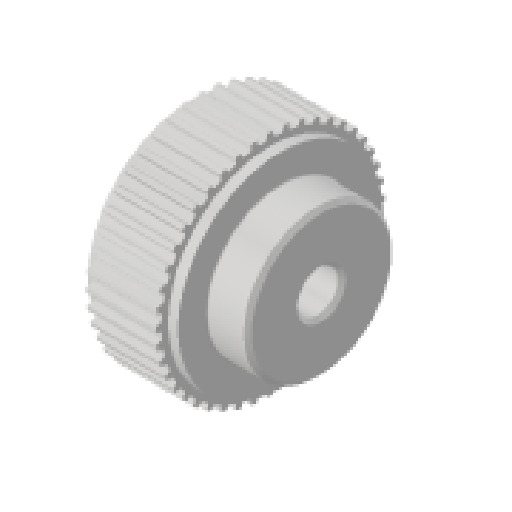
# Autodesk Inventor part: 4202514444
Saved by Autodesk Inventor 2025.1 (Build 291241000, 241)
## iProperties
Category: PARTsolutions
Company: CHIARAVALLI
Created: 2025-04-22
Part Number: 4202514444
Material: Generic
Catalog Web Link: www.cadenas.de
Description: MXL 025 BODY-Timing pulleys with pilot bore
Vendor: CHIARAVALLI
Document SubType Name: Modeling
Designer: psAdmin
Manufacturer: CHIARAVALLI
Mass: 7.09327 g
Surface Area: 28.8164 cm^2
Volume: 7.09327 cm^3
Density: 1 g/cm^3
Appearance: PSOLRGB-175-175-175
PSOL_IDENT_0: {$CADENAS_DATA/23d-libs/chiaravalli/open_transmission/toothed_pulleys/timing_pulleys_with_pilot_bore
PSOL_IDENT_1: /mxl/mxl_025_aluminium.prj},167 {VTYP=3D},{NB=4202514444},{LINA=4202514444},{NN=MXL 025 BODY},{DATE=
PSOL_IDENT_2: 05.08.2024 16:01:07},{GEOMDATE=30.04.2024 10:20:00},{VERSION=},{LINEID=120},{WBVAR=},{WBNUMERIC=}  {
PSOL_IDENT_3: NB=4202514444},{LINA=4202514444},{KT=DUMMY},{CODE=42025144},{TYPE=44 MXL 025},{T=44},{EXEC=1F},{DP=2
PSOL_IDENT_4: 8.46},{DE=27.95},{DF=36},{DM=18},{DM1=-},{F=11.0},{L=16},{D=5},{NF=510},{WEIGHT=0.03},{MAT=Aluminium
PSOL_IDENT_5: 6082-T6},{DX=5},{NFX=510},{DM1X=0.0},{L1=25.0}
NB: 4202514444
NN: MXL 025 BODY
NT: Timing pulleys with pilot bore
NBSYN: $CODE.$T.
LINA: 4202514444
CATALOG: Chiaravalli
CODE: 42025144
T: 44
EXEC: 1F
DP: 28.46
DE: 27.95
DF: 36
DM: 18
DM1: -
F: 11
L: 16
D: 5
NF: 510
WEIGHT: 0.03
MAT: Aluminium 6082-T6
DX: 5
NFX: 510
DM1X: 0
L1: 25
SUPPLIER: CHIARAVALLI
ARTICLENO: 4202514444
BOMINFO: 4202514444
CREATOR: CADENAS GmbH
Title: 4202514444
Author: Cadenas PARTsolutions
Comments: Timing pulleys with pilot bore
Autodesk Inventor part; units mm, degrees
sketch "Sketch_5" plane through (0, 0, 0) normal (0, 0, 1) x (1, 0, 0)
  line L0 (16, 0) -> (0, 0)
  line L1 (0, 3) -> (0.5, 2.5)
  line L2 (0.5, 2.5) -> (15.5, 2.5)
  line L3 (15.5, 2.5) -> (16, 3)
  line L4 (16, 3) -> (16, 8.5)
  line L5 (16, 8.5) -> (15.5, 9)
  line L6 (15.5, 9) -> (11.2, 9)
  arc A0 (11, 9.2) -> (11.2, 9) centre (11.2, 9.2) ccw
  line L7 (11, 9.2) -> (11, 12.5)
  line L8 (11, 12.5) -> (9.75, 12.5)
  line L9 (9.75, 12.5) -> (9.75, 16.77)
  line L10 (9.75, 16.77) -> (1.25, 16.77)
  line L11 (1.25, 16.77) -> (1.25, 12.5)
  line L12 (1.25, 12.5) -> (0, 12.5)
  line L13 (0, 12.5) -> (0, 3)
  constraints: 28 end point, 2 point on circle, 1 centre point
revolve "Revolution1" add sketch "Sketch_5" angle 360 about axis through (16, 0, 0) along (1, 0, 0)
sketch "Sketch_3" plane through (1.25, 0, 0) normal (1, 0, 0) x (0, 0, -1)
  line L0 (-27.95, 27.95) -> (-27.95, -27.95)
  line L1 (-27.95, -27.95) -> (27.95, -27.95)
  line L2 (27.95, -27.95) -> (27.95, 27.95)
  line L3 (27.95, 27.95) -> (-27.95, 27.95)
  arc A0 (-13.973, 0.2355) -> (-13.973, -0.2355) centre (0, 0) ccw
  arc A1 (-13.973, -0.2355) -> (-13.8923, -0.3319) centre (-13.873, -0.2338) ccw
  line L4 (-13.8923, -0.3319) -> (-13.509, -0.4073)
  arc A2 (-13.2673, -0.6862) -> (-13.509, -0.4073) centre (-13.5669, -0.7016) ccw
  arc A3 (-13.2673, -0.6862) -> (-13.2299, -1.209) centre (0, 0) ccw
  arc A4 (-13.4295, -1.5194) -> (-13.2299, -1.209) centre (-13.5286, -1.2363) ccw
  line L5 (-13.4295, -1.5194) -> (-13.7982, -1.6485)
  arc A5 (-13.7982, -1.6485) -> (-13.8643, -1.7555) centre (-13.7651, -1.7429) ccw
  arc A6 (-13.8643, -1.7555) -> (-13.7973, -2.2217) centre (0, 0) ccw
  arc A7 (-13.7973, -2.2217) -> (-13.7037, -2.3056) centre (-13.6985, -2.2058) ccw
  line L6 (-13.7037, -2.3056) -> (-13.3135, -2.3257)
  arc A8 (-13.0346, -2.5673) -> (-13.3135, -2.3257) centre (-13.3289, -2.6253) ccw
  arc A9 (-13.0346, -2.5673) -> (-12.9232, -3.0795) centre (0, 0) ccw
  arc A10 (-13.0765, -3.4151) -> (-12.9232, -3.0795) centre (-13.215, -3.149) ccw
  line L7 (-13.0765, -3.4151) -> (-13.4231, -3.5954)
  arc A11 (-13.4231, -3.5954) -> (-13.4734, -3.7107) centre (-13.3769, -3.6841) ccw
  arc A12 (-13.4734, -3.7107) -> (-13.3407, -4.1626) centre (0, 0) ccw
  arc A13 (-13.3407, -4.1626) -> (-13.2361, -4.2324) centre (-13.2452, -4.1328) ccw
  line L8 (-13.2361, -4.2324) -> (-12.847, -4.1967)
  arc A14 (-12.5365, -4.3962) -> (-12.847, -4.1967) centre (-12.8196, -4.4955) ccw
  arc A15 (-12.5365, -4.3962) -> (-12.3534, -4.8873) centre (0, 0) ccw
  arc A16 (-12.4574, -5.2414) -> (-12.3534, -4.8873) centre (-12.6323, -4.9976) ccw
  line L9 (-12.4574, -5.2414) -> (-12.7748, -5.4691)
  arc A17 (-12.7748, -5.4691) -> (-12.8081, -5.5904) centre (-12.7165, -5.5504) ccw
  arc A18 (-12.8081, -5.5904) -> (-12.6125, -6.0188) centre (0, 0) ccw
  arc A19 (-12.6125, -6.0188) -> (-12.499, -6.073) centre (-12.5222, -5.9757) ccw
  line L10 (-12.499, -6.073) -> (-12.119, -5.9823)
  arc A20 (-11.7833, -6.1356) -> (-12.119, -5.9823) centre (-12.0494, -6.2741) ccw
  arc A21 (-11.7833, -6.1356) -> (-11.5321, -6.5956) centre (0, 0) ccw
  arc A22 (-11.5847, -6.9609) -> (-11.5321, -6.5956) centre (-11.7925, -6.7445) ccw
  line L11 (-11.5847, -6.9609) -> (-11.8664, -7.2315)
  arc A23 (-11.8664, -7.2315) -> (-11.8822, -7.3563) centre (-11.7971, -7.3036) ccw
  arc A24 (-11.8822, -7.3563) -> (-11.6275, -7.7525) centre (0, 0) ccw
  arc A25 (-11.6275, -7.7525) -> (-11.5075, -7.79) centre (-11.5443, -7.697) ccw
  line L12 (-11.5075, -7.79) -> (-11.1443, -7.6461)
  arc A26 (-10.7902, -7.7501) -> (-11.1443, -7.6461) centre (-11.0338, -7.9251) ccw
  arc A27 (-10.7902, -7.7501) -> (-10.4761, -8.1697) centre (0, 0) ccw
  arc A28 (-10.4761, -8.5387) -> (-10.4761, -8.1697) centre (-10.7126, -8.3541) ccw
  line L13 (-10.4761, -8.5387) -> (-10.7165, -8.8467)
  arc A29 (-10.7165, -8.8467) -> (-10.7143, -8.9724) centre (-10.6376, -8.9082) ccw
  arc A30 (-10.7143, -8.9724) -> (-10.4059, -9.3284) centre (0, 0) ccw
  arc A31 (-10.4059, -9.3284) -> (-10.2817, -9.3484) centre (-10.3314, -9.2616) ccw
  line L14 (-10.2817, -9.3484) -> (-9.9427, -9.1543)
  arc A32 (-9.5774, -9.2068) -> (-9.9427, -9.1543) centre (-9.7937, -9.4147) ccw
  arc A33 (-9.5774, -9.2068) -> (-9.2068, -9.5774) centre (0, 0) ccw
  arc A34 (-9.1543, -9.9427) -> (-9.2068, -9.5774) centre (-9.4147, -9.7937) ccw
  line L15 (-9.1543, -9.9427) -> (-9.3484, -10.2817)
  arc A35 (-9.3484, -10.2817) -> (-9.3284, -10.4059) centre (-9.2616, -10.3314) ccw
  arc A36 (-9.3284, -10.4059) -> (-8.9724, -10.7143) centre (0, 0) ccw
  arc A37 (-8.9724, -10.7143) -> (-8.8467, -10.7165) centre (-8.9082, -10.6376) ccw
  line L16 (-8.8467, -10.7165) -> (-8.5387, -10.4761)
  arc A38 (-8.1697, -10.4761) -> (-8.5387, -10.4761) centre (-8.3541, -10.7126) ccw
  arc A39 (-8.1697, -10.4761) -> (-7.7501, -10.7902) centre (0, 0) ccw
  arc A40 (-7.6461, -11.1443) -> (-7.7501, -10.7902) centre (-7.9251, -11.0338) ccw
  line L17 (-7.6461, -11.1443) -> (-7.79, -11.5075)
  arc A41 (-7.79, -11.5075) -> (-7.7525, -11.6275) centre (-7.697, -11.5443) ccw
  arc A42 (-7.7525, -11.6275) -> (-7.3563, -11.8822) centre (0, 0) ccw
  arc A43 (-7.3563, -11.8822) -> (-7.2315, -11.8664) centre (-7.3036, -11.7971) ccw
  line L18 (-7.2315, -11.8664) -> (-6.9609, -11.5847)
  arc A44 (-6.5956, -11.5321) -> (-6.9609, -11.5847) centre (-6.7445, -11.7925) ccw
  arc A45 (-6.5956, -11.5321) -> (-6.1356, -11.7833) centre (0, 0) ccw
  arc A46 (-5.9823, -12.119) -> (-6.1356, -11.7833) centre (-6.2741, -12.0494) ccw
  line L19 (-5.9823, -12.119) -> (-6.073, -12.499)
  arc A47 (-6.073, -12.499) -> (-6.0188, -12.6125) centre (-5.9757, -12.5222) ccw
  arc A48 (-6.0188, -12.6125) -> (-5.5904, -12.8081) centre (0, 0) ccw
  arc A49 (-5.5904, -12.8081) -> (-5.4691, -12.7748) centre (-5.5504, -12.7165) ccw
  line L20 (-5.4691, -12.7748) -> (-5.2414, -12.4574)
  arc A50 (-4.8873, -12.3534) -> (-5.2414, -12.4574) centre (-4.9976, -12.6323) ccw
  arc A51 (-4.8873, -12.3534) -> (-4.3962, -12.5365) centre (0, 0) ccw
  arc A52 (-4.1967, -12.847) -> (-4.3962, -12.5365) centre (-4.4955, -12.8196) ccw
  line L21 (-4.1967, -12.847) -> (-4.2324, -13.2361)
  arc A53 (-4.2324, -13.2361) -> (-4.1626, -13.3407) centre (-4.1328, -13.2452) ccw
  arc A54 (-4.1626, -13.3407) -> (-3.7107, -13.4734) centre (0, 0) ccw
  arc A55 (-3.7107, -13.4734) -> (-3.5954, -13.4231) centre (-3.6841, -13.3769) ccw
  line L22 (-3.5954, -13.4231) -> (-3.4151, -13.0765)
  arc A56 (-3.0795, -12.9232) -> (-3.4151, -13.0765) centre (-3.149, -13.215) ccw
  arc A57 (-3.0795, -12.9232) -> (-2.5673, -13.0346) centre (0, 0) ccw
  arc A58 (-2.3257, -13.3135) -> (-2.5673, -13.0346) centre (-2.6253, -13.3289) ccw
  line L23 (-2.3257, -13.3135) -> (-2.3056, -13.7037)
  arc A59 (-2.3056, -13.7037) -> (-2.2217, -13.7973) centre (-2.2058, -13.6985) ccw
  arc A60 (-2.2217, -13.7973) -> (-1.7555, -13.8643) centre (0, 0) ccw
  arc A61 (-1.7555, -13.8643) -> (-1.6485, -13.7982) centre (-1.7429, -13.7651) ccw
  line L24 (-1.6485, -13.7982) -> (-1.5194, -13.4295)
  arc A62 (-1.209, -13.2299) -> (-1.5194, -13.4295) centre (-1.2363, -13.5286) ccw
  arc A63 (-1.209, -13.2299) -> (-0.6862, -13.2673) centre (0, 0) ccw
  arc A64 (-0.4073, -13.509) -> (-0.6862, -13.2673) centre (-0.7016, -13.5669) ccw
  line L25 (-0.4073, -13.509) -> (-0.3319, -13.8923)
  arc A65 (-0.3319, -13.8923) -> (-0.2355, -13.973) centre (-0.2338, -13.873) ccw
  arc A66 (-0.2355, -13.973) -> (0.2355, -13.973) centre (0, 0) ccw
  arc A67 (0.2355, -13.973) -> (0.3319, -13.8923) centre (0.2338, -13.873) ccw
  line L26 (0.3319, -13.8923) -> (0.4073, -13.509)
  arc A68 (0.6862, -13.2673) -> (0.4073, -13.509) centre (0.7016, -13.5669) ccw
  arc A69 (0.6862, -13.2673) -> (1.209, -13.2299) centre (0, 0) ccw
  arc A70 (1.5194, -13.4295) -> (1.209, -13.2299) centre (1.2363, -13.5286) ccw
  line L27 (1.5194, -13.4295) -> (1.6485, -13.7982)
  arc A71 (1.6485, -13.7982) -> (1.7555, -13.8643) centre (1.7429, -13.7651) ccw
  arc A72 (1.7555, -13.8643) -> (2.2217, -13.7973) centre (0, 0) ccw
  arc A73 (2.2217, -13.7973) -> (2.3056, -13.7037) centre (2.2058, -13.6985) ccw
  line L28 (2.3056, -13.7037) -> (2.3257, -13.3135)
  arc A74 (2.5673, -13.0346) -> (2.3257, -13.3135) centre (2.6253, -13.3289) ccw
  arc A75 (2.5673, -13.0346) -> (3.0795, -12.9232) centre (0, 0) ccw
  arc A76 (3.4151, -13.0765) -> (3.0795, -12.9232) centre (3.149, -13.215) ccw
  line L29 (3.4151, -13.0765) -> (3.5954, -13.4231)
  arc A77 (3.5954, -13.4231) -> (3.7107, -13.4734) centre (3.6841, -13.3769) ccw
  arc A78 (3.7107, -13.4734) -> (4.1626, -13.3407) centre (0, 0) ccw
  arc A79 (4.1626, -13.3407) -> (4.2324, -13.2361) centre (4.1328, -13.2452) ccw
  line L30 (4.2324, -13.2361) -> (4.1967, -12.847)
  arc A80 (4.3962, -12.5365) -> (4.1967, -12.847) centre (4.4955, -12.8196) ccw
  arc A81 (4.3962, -12.5365) -> (4.8873, -12.3534) centre (0, 0) ccw
  arc A82 (5.2414, -12.4574) -> (4.8873, -12.3534) centre (4.9976, -12.6323) ccw
  line L31 (5.2414, -12.4574) -> (5.4691, -12.7748)
  arc A83 (5.4691, -12.7748) -> (5.5904, -12.8081) centre (5.5504, -12.7165) ccw
  arc A84 (5.5904, -12.8081) -> (6.0188, -12.6125) centre (0, 0) ccw
  arc A85 (6.0188, -12.6125) -> (6.073, -12.499) centre (5.9757, -12.5222) ccw
  line L32 (6.073, -12.499) -> (5.9823, -12.119)
  arc A86 (6.1356, -11.7833) -> (5.9823, -12.119) centre (6.2741, -12.0494) ccw
  arc A87 (6.1356, -11.7833) -> (6.5956, -11.5321) centre (0, 0) ccw
  arc A88 (6.9609, -11.5847) -> (6.5956, -11.5321) centre (6.7445, -11.7925) ccw
  line L33 (6.9609, -11.5847) -> (7.2315, -11.8664)
  arc A89 (7.2315, -11.8664) -> (7.3563, -11.8822) centre (7.3036, -11.7971) ccw
  arc A90 (7.3563, -11.8822) -> (7.7525, -11.6275) centre (0, 0) ccw
  arc A91 (7.7525, -11.6275) -> (7.79, -11.5075) centre (7.697, -11.5443) ccw
  line L34 (7.79, -11.5075) -> (7.6461, -11.1443)
  arc A92 (7.7501, -10.7902) -> (7.6461, -11.1443) centre (7.9251, -11.0338) ccw
  arc A93 (7.7501, -10.7902) -> (8.1697, -10.4761) centre (0, 0) ccw
  arc A94 (8.5387, -10.4761) -> (8.1697, -10.4761) centre (8.3541, -10.7126) ccw
  line L35 (8.5387, -10.4761) -> (8.8467, -10.7165)
  arc A95 (8.8467, -10.7165) -> (8.9724, -10.7143) centre (8.9082, -10.6376) ccw
  arc A96 (8.9724, -10.7143) -> (9.3284, -10.4059) centre (0, 0) ccw
  arc A97 (9.3284, -10.4059) -> (9.3484, -10.2817) centre (9.2616, -10.3314) ccw
  line L36 (9.3484, -10.2817) -> (9.1543, -9.9427)
  arc A98 (9.2068, -9.5774) -> (9.1543, -9.9427) centre (9.4147, -9.7937) ccw
  arc A99 (9.2068, -9.5774) -> (9.5774, -9.2068) centre (0, 0) ccw
  arc A100 (9.9427, -9.1543) -> (9.5774, -9.2068) centre (9.7937, -9.4147) ccw
  line L37 (9.9427, -9.1543) -> (10.2817, -9.3484)
  arc A101 (10.2817, -9.3484) -> (10.4059, -9.3284) centre (10.3314, -9.2616) ccw
  arc A102 (10.4059, -9.3284) -> (10.7143, -8.9724) centre (0, 0) ccw
  arc A103 (10.7143, -8.9724) -> (10.7165, -8.8467) centre (10.6376, -8.9082) ccw
  line L38 (10.7165, -8.8467) -> (10.4761, -8.5387)
  arc A104 (10.4761, -8.1697) -> (10.4761, -8.5387) centre (10.7126, -8.3541) ccw
  arc A105 (10.4761, -8.1697) -> (10.7902, -7.7501) centre (0, 0) ccw
  arc A106 (11.1443, -7.6461) -> (10.7902, -7.7501) centre (11.0338, -7.9251) ccw
  line L39 (11.1443, -7.6461) -> (11.5075, -7.79)
  arc A107 (11.5075, -7.79) -> (11.6275, -7.7525) centre (11.5443, -7.697) ccw
  arc A108 (11.6275, -7.7525) -> (11.8822, -7.3563) centre (0, 0) ccw
  arc A109 (11.8822, -7.3563) -> (11.8664, -7.2315) centre (11.7971, -7.3036) ccw
  line L40 (11.8664, -7.2315) -> (11.5847, -6.9609)
  arc A110 (11.5321, -6.5956) -> (11.5847, -6.9609) centre (11.7925, -6.7445) ccw
  arc A111 (11.5321, -6.5956) -> (11.7833, -6.1356) centre (0, 0) ccw
  arc A112 (12.119, -5.9823) -> (11.7833, -6.1356) centre (12.0494, -6.2741) ccw
  line L41 (12.119, -5.9823) -> (12.499, -6.073)
  arc A113 (12.499, -6.073) -> (12.6125, -6.0188) centre (12.5222, -5.9757) ccw
  arc A114 (12.6125, -6.0188) -> (12.8081, -5.5904) centre (0, 0) ccw
  arc A115 (12.8081, -5.5904) -> (12.7748, -5.4691) centre (12.7165, -5.5504) ccw
  line L42 (12.7748, -5.4691) -> (12.4574, -5.2414)
  arc A116 (12.3534, -4.8873) -> (12.4574, -5.2414) centre (12.6323, -4.9976) ccw
  arc A117 (12.3534, -4.8873) -> (12.5365, -4.3962) centre (0, 0) ccw
  arc A118 (12.847, -4.1967) -> (12.5365, -4.3962) centre (12.8196, -4.4955) ccw
  line L43 (12.847, -4.1967) -> (13.2361, -4.2324)
  arc A119 (13.2361, -4.2324) -> (13.3407, -4.1626) centre (13.2452, -4.1328) ccw
  arc A120 (13.3407, -4.1626) -> (13.4734, -3.7107) centre (0, 0) ccw
  arc A121 (13.4734, -3.7107) -> (13.4231, -3.5954) centre (13.3769, -3.6841) ccw
  line L44 (13.4231, -3.5954) -> (13.0765, -3.4151)
  arc A122 (12.9232, -3.0795) -> (13.0765, -3.4151) centre (13.215, -3.149) ccw
  arc A123 (12.9232, -3.0795) -> (13.0346, -2.5673) centre (0, 0) ccw
  arc A124 (13.3135, -2.3257) -> (13.0346, -2.5673) centre (13.3289, -2.6253) ccw
  line L45 (13.3135, -2.3257) -> (13.7037, -2.3056)
  arc A125 (13.7037, -2.3056) -> (13.7973, -2.2217) centre (13.6985, -2.2058) ccw
  arc A126 (13.7973, -2.2217) -> (13.8643, -1.7555) centre (0, 0) ccw
  arc A127 (13.8643, -1.7555) -> (13.7982, -1.6485) centre (13.7651, -1.7429) ccw
  line L46 (13.7982, -1.6485) -> (13.4295, -1.5194)
  arc A128 (13.2299, -1.209) -> (13.4295, -1.5194) centre (13.5286, -1.2363) ccw
  arc A129 (13.2299, -1.209) -> (13.2673, -0.6862) centre (0, 0) ccw
  arc A130 (13.509, -0.4073) -> (13.2673, -0.6862) centre (13.5669, -0.7016) ccw
  line L47 (13.509, -0.4073) -> (13.8923, -0.3319)
  arc A131 (13.8923, -0.3319) -> (13.973, -0.2355) centre (13.873, -0.2338) ccw
  arc A132 (13.973, -0.2355) -> (13.973, 0.2355) centre (0, 0) ccw
  arc A133 (13.973, 0.2355) -> (13.8923, 0.3319) centre (13.873, 0.2338) ccw
  line L48 (13.8923, 0.3319) -> (13.509, 0.4073)
  arc A134 (13.2673, 0.6862) -> (13.509, 0.4073) centre (13.5669, 0.7016) ccw
  arc A135 (13.2673, 0.6862) -> (13.2299, 1.209) centre (0, 0) ccw
  arc A136 (13.4295, 1.5194) -> (13.2299, 1.209) centre (13.5286, 1.2363) ccw
  line L49 (13.4295, 1.5194) -> (13.7982, 1.6485)
  arc A137 (13.7982, 1.6485) -> (13.8643, 1.7555) centre (13.7651, 1.7429) ccw
  arc A138 (13.8643, 1.7555) -> (13.7973, 2.2217) centre (0, 0) ccw
  arc A139 (13.7973, 2.2217) -> (13.7037, 2.3056) centre (13.6985, 2.2058) ccw
  line L50 (13.7037, 2.3056) -> (13.3135, 2.3257)
  arc A140 (13.0346, 2.5673) -> (13.3135, 2.3257) centre (13.3289, 2.6253) ccw
  arc A141 (13.0346, 2.5673) -> (12.9232, 3.0795) centre (0, 0) ccw
  arc A142 (13.0765, 3.4151) -> (12.9232, 3.0795) centre (13.215, 3.149) ccw
  line L51 (13.0765, 3.4151) -> (13.4231, 3.5954)
  arc A143 (13.4231, 3.5954) -> (13.4734, 3.7107) centre (13.3769, 3.6841) ccw
  arc A144 (13.4734, 3.7107) -> (13.3407, 4.1626) centre (0, 0) ccw
  arc A145 (13.3407, 4.1626) -> (13.2361, 4.2324) centre (13.2452, 4.1328) ccw
  line L52 (13.2361, 4.2324) -> (12.847, 4.1967)
  arc A146 (12.5365, 4.3962) -> (12.847, 4.1967) centre (12.8196, 4.4955) ccw
  arc A147 (12.5365, 4.3962) -> (12.3534, 4.8873) centre (0, 0) ccw
  arc A148 (12.4574, 5.2414) -> (12.3534, 4.8873) centre (12.6323, 4.9976) ccw
  line L53 (12.4574, 5.2414) -> (12.7748, 5.4691)
  arc A149 (12.7748, 5.4691) -> (12.8081, 5.5904) centre (12.7165, 5.5504) ccw
  arc A150 (12.8081, 5.5904) -> (12.6125, 6.0188) centre (0, 0) ccw
  arc A151 (12.6125, 6.0188) -> (12.499, 6.073) centre (12.5222, 5.9757) ccw
  line L54 (12.499, 6.073) -> (12.119, 5.9823)
  arc A152 (11.7833, 6.1356) -> (12.119, 5.9823) centre (12.0494, 6.2741) ccw
  arc A153 (11.7833, 6.1356) -> (11.5321, 6.5956) centre (0, 0) ccw
  arc A154 (11.5847, 6.9609) -> (11.5321, 6.5956) centre (11.7925, 6.7445) ccw
  line L55 (11.5847, 6.9609) -> (11.8664, 7.2315)
  arc A155 (11.8664, 7.2315) -> (11.8822, 7.3563) centre (11.7971, 7.3036) ccw
  arc A156 (11.8822, 7.3563) -> (11.6275, 7.7525) centre (0, 0) ccw
  arc A157 (11.6275, 7.7525) -> (11.5075, 7.79) centre (11.5443, 7.697) ccw
  line L56 (11.5075, 7.79) -> (11.1443, 7.6461)
  arc A158 (10.7902, 7.7501) -> (11.1443, 7.6461) centre (11.0338, 7.9251) ccw
  arc A159 (10.7902, 7.7501) -> (10.4761, 8.1697) centre (0, 0) ccw
  arc A160 (10.4761, 8.5387) -> (10.4761, 8.1697) centre (10.7126, 8.3541) ccw
  line L57 (10.4761, 8.5387) -> (10.7165, 8.8467)
  arc A161 (10.7165, 8.8467) -> (10.7143, 8.9724) centre (10.6376, 8.9082) ccw
  arc A162 (10.7143, 8.9724) -> (10.4059, 9.3284) centre (0, 0) ccw
  arc A163 (10.4059, 9.3284) -> (10.2817, 9.3484) centre (10.3314, 9.2616) ccw
  line L58 (10.2817, 9.3484) -> (9.9427, 9.1543)
  arc A164 (9.5774, 9.2068) -> (9.9427, 9.1543) centre (9.7937, 9.4147) ccw
  arc A165 (9.5774, 9.2068) -> (9.2068, 9.5774) centre (0, 0) ccw
  arc A166 (9.1543, 9.9427) -> (9.2068, 9.5774) centre (9.4147, 9.7937) ccw
  line L59 (9.1543, 9.9427) -> (9.3484, 10.2817)
  arc A167 (9.3484, 10.2817) -> (9.3284, 10.4059) centre (9.2616, 10.3314) ccw
  arc A168 (9.3284, 10.4059) -> (8.9724, 10.7143) centre (0, 0) ccw
  arc A169 (8.9724, 10.7143) -> (8.8467, 10.7165) centre (8.9082, 10.6376) ccw
  line L60 (8.8467, 10.7165) -> (8.5387, 10.4761)
  arc A170 (8.1697, 10.4761) -> (8.5387, 10.4761) centre (8.3541, 10.7126) ccw
  arc A171 (8.1697, 10.4761) -> (7.7501, 10.7902) centre (0, 0) ccw
  arc A172 (7.6461, 11.1443) -> (7.7501, 10.7902) centre (7.9251, 11.0338) ccw
  line L61 (7.6461, 11.1443) -> (7.79, 11.5075)
  arc A173 (7.79, 11.5075) -> (7.7525, 11.6275) centre (7.697, 11.5443) ccw
  arc A174 (7.7525, 11.6275) -> (7.3563, 11.8822) centre (0, 0) ccw
  arc A175 (7.3563, 11.8822) -> (7.2315, 11.8664) centre (7.3036, 11.7971) ccw
  line L62 (7.2315, 11.8664) -> (6.9609, 11.5847)
  arc A176 (6.5956, 11.5321) -> (6.9609, 11.5847) centre (6.7445, 11.7925) ccw
  arc A177 (6.5956, 11.5321) -> (6.1356, 11.7833) centre (0, 0) ccw
  arc A178 (5.9823, 12.119) -> (6.1356, 11.7833) centre (6.2741, 12.0494) ccw
  line L63 (5.9823, 12.119) -> (6.073, 12.499)
  arc A179 (6.073, 12.499) -> (6.0188, 12.6125) centre (5.9757, 12.5222) ccw
  arc A180 (6.0188, 12.6125) -> (5.5904, 12.8081) centre (0, 0) ccw
  arc A181 (5.5904, 12.8081) -> (5.4691, 12.7748) centre (5.5504, 12.7165) ccw
  line L64 (5.4691, 12.7748) -> (5.2414, 12.4574)
  arc A182 (4.8873, 12.3534) -> (5.2414, 12.4574) centre (4.9976, 12.6323) ccw
  arc A183 (4.8873, 12.3534) -> (4.3962, 12.5365) centre (0, 0) ccw
  arc A184 (4.1967, 12.847) -> (4.3962, 12.5365) centre (4.4955, 12.8196) ccw
  line L65 (4.1967, 12.847) -> (4.2324, 13.2361)
  arc A185 (4.2324, 13.2361) -> (4.1626, 13.3407) centre (4.1328, 13.2452) ccw
  arc A186 (4.1626, 13.3407) -> (3.7107, 13.4734) centre (0, 0) ccw
  arc A187 (3.7107, 13.4734) -> (3.5954, 13.4231) centre (3.6841, 13.3769) ccw
  line L66 (3.5954, 13.4231) -> (3.4151, 13.0765)
  arc A188 (3.0795, 12.9232) -> (3.4151, 13.0765) centre (3.149, 13.215) ccw
  arc A189 (3.0795, 12.9232) -> (2.5673, 13.0346) centre (0, 0) ccw
  arc A190 (2.3257, 13.3135) -> (2.5673, 13.0346) centre (2.6253, 13.3289) ccw
  line L67 (2.3257, 13.3135) -> (2.3056, 13.7037)
  arc A191 (2.3056, 13.7037) -> (2.2217, 13.7973) centre (2.2058, 13.6985) ccw
  arc A192 (2.2217, 13.7973) -> (1.7555, 13.8643) centre (0, 0) ccw
  arc A193 (1.7555, 13.8643) -> (1.6485, 13.7982) centre (1.7429, 13.7651) ccw
  line L68 (1.6485, 13.7982) -> (1.5194, 13.4295)
  arc A194 (1.209, 13.2299) -> (1.5194, 13.4295) centre (1.2363, 13.5286) ccw
  arc A195 (1.209, 13.2299) -> (0.6862, 13.2673) centre (0, 0) ccw
  arc A196 (0.4073, 13.509) -> (0.6862, 13.2673) centre (0.7016, 13.5669) ccw
  line L69 (0.4073, 13.509) -> (0.3319, 13.8923)
  arc A197 (0.3319, 13.8923) -> (0.2355, 13.973) centre (0.2338, 13.873) ccw
  arc A198 (0.2355, 13.973) -> (-0.2355, 13.973) centre (0, 0) ccw
  arc A199 (-0.2355, 13.973) -> (-0.3319, 13.8923) centre (-0.2338, 13.873) ccw
  line L70 (-0.3319, 13.8923) -> (-0.4073, 13.509)
  arc A200 (-0.6862, 13.2673) -> (-0.4073, 13.509) centre (-0.7016, 13.5669) ccw
  arc A201 (-0.6862, 13.2673) -> (-1.209, 13.2299) centre (0, 0) ccw
  arc A202 (-1.5194, 13.4295) -> (-1.209, 13.2299) centre (-1.2363, 13.5286) ccw
  line L71 (-1.5194, 13.4295) -> (-1.6485, 13.7982)
  arc A203 (-1.6485, 13.7982) -> (-1.7555, 13.8643) centre (-1.7429, 13.7651) ccw
  arc A204 (-1.7555, 13.8643) -> (-2.2217, 13.7973) centre (0, 0) ccw
  arc A205 (-2.2217, 13.7973) -> (-2.3056, 13.7037) centre (-2.2058, 13.6985) ccw
  line L72 (-2.3056, 13.7037) -> (-2.3257, 13.3135)
  arc A206 (-2.5673, 13.0346) -> (-2.3257, 13.3135) centre (-2.6253, 13.3289) ccw
  arc A207 (-2.5673, 13.0346) -> (-3.0795, 12.9232) centre (0, 0) ccw
  arc A208 (-3.4151, 13.0765) -> (-3.0795, 12.9232) centre (-3.149, 13.215) ccw
  line L73 (-3.4151, 13.0765) -> (-3.5954, 13.4231)
  arc A209 (-3.5954, 13.4231) -> (-3.7107, 13.4734) centre (-3.6841, 13.3769) ccw
  arc A210 (-3.7107, 13.4734) -> (-4.1626, 13.3407) centre (0, 0) ccw
  arc A211 (-4.1626, 13.3407) -> (-4.2324, 13.2361) centre (-4.1328, 13.2452) ccw
  line L74 (-4.2324, 13.2361) -> (-4.1967, 12.847)
  arc A212 (-4.3962, 12.5365) -> (-4.1967, 12.847) centre (-4.4955, 12.8196) ccw
  arc A213 (-4.3962, 12.5365) -> (-4.8873, 12.3534) centre (0, 0) ccw
  arc A214 (-5.2414, 12.4574) -> (-4.8873, 12.3534) centre (-4.9976, 12.6323) ccw
  line L75 (-5.2414, 12.4574) -> (-5.4691, 12.7748)
  arc A215 (-5.4691, 12.7748) -> (-5.5904, 12.8081) centre (-5.5504, 12.7165) ccw
  arc A216 (-5.5904, 12.8081) -> (-6.0188, 12.6125) centre (0, 0) ccw
  arc A217 (-6.0188, 12.6125) -> (-6.073, 12.499) centre (-5.9757, 12.5222) ccw
  line L76 (-6.073, 12.499) -> (-5.9823, 12.119)
  arc A218 (-6.1356, 11.7833) -> (-5.9823, 12.119) centre (-6.2741, 12.0494) ccw
  arc A219 (-6.1356, 11.7833) -> (-6.5956, 11.5321) centre (0, 0) ccw
  arc A220 (-6.9609, 11.5847) -> (-6.5956, 11.5321) centre (-6.7445, 11.7925) ccw
  line L77 (-6.9609, 11.5847) -> (-7.2315, 11.8664)
  arc A221 (-7.2315, 11.8664) -> (-7.3563, 11.8822) centre (-7.3036, 11.7971) ccw
  arc A222 (-7.3563, 11.8822) -> (-7.7525, 11.6275) centre (0, 0) ccw
  arc A223 (-7.7525, 11.6275) -> (-7.79, 11.5075) centre (-7.697, 11.5443) ccw
  line L78 (-7.79, 11.5075) -> (-7.6461, 11.1443)
  arc A224 (-7.7501, 10.7902) -> (-7.6461, 11.1443) centre (-7.9251, 11.0338) ccw
  arc A225 (-7.7501, 10.7902) -> (-8.1697, 10.4761) centre (0, 0) ccw
  arc A226 (-8.5387, 10.4761) -> (-8.1697, 10.4761) centre (-8.3541, 10.7126) ccw
  line L79 (-8.5387, 10.4761) -> (-8.8467, 10.7165)
  arc A227 (-8.8467, 10.7165) -> (-8.9724, 10.7143) centre (-8.9082, 10.6376) ccw
  arc A228 (-8.9724, 10.7143) -> (-9.3284, 10.4059) centre (0, 0) ccw
  arc A229 (-9.3284, 10.4059) -> (-9.3484, 10.2817) centre (-9.2616, 10.3314) ccw
  line L80 (-9.3484, 10.2817) -> (-9.1543, 9.9427)
  arc A230 (-9.2068, 9.5774) -> (-9.1543, 9.9427) centre (-9.4147, 9.7937) ccw
  arc A231 (-9.2068, 9.5774) -> (-9.5774, 9.2068) centre (0, 0) ccw
  arc A232 (-9.9427, 9.1543) -> (-9.5774, 9.2068) centre (-9.7937, 9.4147) ccw
  line L81 (-9.9427, 9.1543) -> (-10.2817, 9.3484)
  arc A233 (-10.2817, 9.3484) -> (-10.4059, 9.3284) centre (-10.3314, 9.2616) ccw
  arc A234 (-10.4059, 9.3284) -> (-10.7143, 8.9724) centre (0, 0) ccw
  arc A235 (-10.7143, 8.9724) -> (-10.7165, 8.8467) centre (-10.6376, 8.9082) ccw
  line L82 (-10.7165, 8.8467) -> (-10.4761, 8.5387)
  arc A236 (-10.4761, 8.1697) -> (-10.4761, 8.5387) centre (-10.7126, 8.3541) ccw
  arc A237 (-10.4761, 8.1697) -> (-10.7902, 7.7501) centre (0, 0) ccw
  arc A238 (-11.1443, 7.6461) -> (-10.7902, 7.7501) centre (-11.0338, 7.9251) ccw
  line L83 (-11.1443, 7.6461) -> (-11.5075, 7.79)
  arc A239 (-11.5075, 7.79) -> (-11.6275, 7.7525) centre (-11.5443, 7.697) ccw
  arc A240 (-11.6275, 7.7525) -> (-11.8822, 7.3563) centre (0, 0) ccw
  arc A241 (-11.8822, 7.3563) -> (-11.8664, 7.2315) centre (-11.7971, 7.3036) ccw
  line L84 (-11.8664, 7.2315) -> (-11.5847, 6.9609)
  arc A242 (-11.5321, 6.5956) -> (-11.5847, 6.9609) centre (-11.7925, 6.7445) ccw
  arc A243 (-11.5321, 6.5956) -> (-11.7833, 6.1356) centre (0, 0) ccw
  arc A244 (-12.119, 5.9823) -> (-11.7833, 6.1356) centre (-12.0494, 6.2741) ccw
  line L85 (-12.119, 5.9823) -> (-12.499, 6.073)
  arc A245 (-12.499, 6.073) -> (-12.6125, 6.0188) centre (-12.5222, 5.9757) ccw
  arc A246 (-12.6125, 6.0188) -> (-12.8081, 5.5904) centre (0, 0) ccw
  arc A247 (-12.8081, 5.5904) -> (-12.7748, 5.4691) centre (-12.7165, 5.5504) ccw
  line L86 (-12.7748, 5.4691) -> (-12.4574, 5.2414)
  arc A248 (-12.3534, 4.8873) -> (-12.4574, 5.2414) centre (-12.6323, 4.9976) ccw
  arc A249 (-12.3534, 4.8873) -> (-12.5365, 4.3962) centre (0, 0) ccw
  arc A250 (-12.847, 4.1967) -> (-12.5365, 4.3962) centre (-12.8196, 4.4955) ccw
  line L87 (-12.847, 4.1967) -> (-13.2361, 4.2324)
  arc A251 (-13.2361, 4.2324) -> (-13.3407, 4.1626) centre (-13.2452, 4.1328) ccw
  arc A252 (-13.3407, 4.1626) -> (-13.4734, 3.7107) centre (0, 0) ccw
  arc A253 (-13.4734, 3.7107) -> (-13.4231, 3.5954) centre (-13.3769, 3.6841) ccw
  line L88 (-13.4231, 3.5954) -> (-13.0765, 3.4151)
  arc A254 (-12.9232, 3.0795) -> (-13.0765, 3.4151) centre (-13.215, 3.149) ccw
  arc A255 (-12.9232, 3.0795) -> (-13.0346, 2.5673) centre (0, 0) ccw
  arc A256 (-13.3135, 2.3257) -> (-13.0346, 2.5673) centre (-13.3289, 2.6253) ccw
  line L89 (-13.3135, 2.3257) -> (-13.7037, 2.3056)
  arc A257 (-13.7037, 2.3056) -> (-13.7973, 2.2217) centre (-13.6985, 2.2058) ccw
  arc A258 (-13.7973, 2.2217) -> (-13.8643, 1.7555) centre (0, 0) ccw
  arc A259 (-13.8643, 1.7555) -> (-13.7982, 1.6485) centre (-13.7651, 1.7429) ccw
  line L90 (-13.7982, 1.6485) -> (-13.4295, 1.5194)
  arc A260 (-13.2299, 1.209) -> (-13.4295, 1.5194) centre (-13.5286, 1.2363) ccw
  arc A261 (-13.2299, 1.209) -> (-13.2673, 0.6862) centre (0, 0) ccw
  arc A262 (-13.509, 0.4073) -> (-13.2673, 0.6862) centre (-13.5669, 0.7016) ccw
  line L91 (-13.509, 0.4073) -> (-13.8923, 0.3319)
  arc A263 (-13.8923, 0.3319) -> (-13.973, 0.2355) centre (-13.873, 0.2338) ccw
  constraints: 528 point on circle, 264 centre point, 184 end point
extrude "Extrusion1" cut sketch "Sketch_3" along normal blind 11
ref_plane "FLL_XY" through (1.25, 0, 0) normal (-1, 0, 0) x (0, 0, -1)
ref_plane "FLL_YZ" through (1.25, 0, 0) normal (0, 0, -1) x (0, -1, 0)
ref_plane "FLL_ZX" through (1.25, 0, 0) normal (0, -1, 0) x (-1, 0, 0)
ref_plane "FLR_XY" through (9.75, 0, 0) normal (1, 0, 0) x (0, 0, -1)
ref_plane "FLR_YZ" through (9.75, 0, 0) normal (0, 0, -1) x (0, 1, 0)
ref_plane "FLR_ZX" through (9.75, 0, 0) normal (0, 1, 0) x (1, 0, 0)
ref_plane "MXL025_D_XY" through (0, 0, 0) normal (-1, 0, 0) x (0, 0, -1)
ref_plane "MXL025_D_YZ" through (0, 0, 0) normal (0, 0, -1) x (0, -1, 0)
ref_plane "MXL025_D_ZX" through (0, 0, 0) normal (0, -1, 0) x (-1, 0, 0)
body "Solid1"
